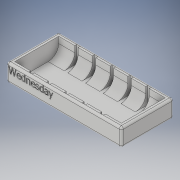
# Autodesk Inventor part: Wednesday
Saved by Autodesk Inventor 2019.4 (Build 234330000, 330)
## iProperties
Created: 2020-10-20
Part Number: Wednesday
Material: Generic
Document SubType Name: Modeling
Designer: daanswinters
Density: 1 g/cm^3
Appearance: Default
Author: daanswinters
Autodesk Inventor part; units mm, degrees
ref_plane "YZ Plane" through (0, 0, 0) normal (1, 0, 0) x (0, 1, 0)
ref_plane "XZ Plane" through (0, 0, 0) normal (0, 1, 0) x (-1, 0, 0)
ref_plane "XY Plane" through (0, 0, 0) normal (0, 0, 1) x (1, 0, 0)
sketch "Sketch1" plane through (0, 0, 0) normal (0, 0, 1) x (1, 0, 0)
  line L0 (55, -8.5) -> (-55, -8.5)
  line L1 (-55, -8.5) -> (-55, 8.5)
  line L2 (-55, 8.5) -> (55, 8.5)
  line L3 (55, 8.5) -> (55, -8.5)
  line L4 (55, -8.5) -> (-55, 8.5) construction
  line L5 (-55, -8.5) -> (55, 8.5) construction
  point P0 (0, 0)
  dimension "d0" = 110
  dimension "d1" = 17
  constraints: 12 end point, 2 midpoint, 2 parallel, 1 horizontal, 1 perpendicular
  measures "d0" distance of L1.end L2.end
  measures "d1" distance of L0.end L1.end
extrude "Extrusion1" add sketch "Sketch1" along normal blind 50
sketch "Sketch2" plane through (-55, 8.5, 0) normal (0, 1, 0) x (1, 0, 0)
  line L0 (0, 0) -> (0, -50) projected
  line L1 (110, -50) -> (0, -50)
  line L2 (0, -50) -> (0, 0)
  line L3 (0, 0) -> (110, 0)
  line L4 (110, 0) -> (110, -50)
  line L5 (110, -50) -> (0, 0) construction
  line L6 (0, -50) -> (110, 0) construction
  line L7 (106, -46) -> (106, -4)
  line L8 (4, -4) -> (4, -46)
  line L9 (56.15, -2) -> (53.85, -2)
  line L10 (53.85, -48) -> (56.15, -48)
  line L11 (56.15, -2) -> (53.85, -48) construction
  line L12 (53.85, -2) -> (56.15, -48) construction
  line L13 (73.15, -2) -> (70.85, -2)
  line L14 (70.85, -48) -> (73.15, -48)
  line L15 (73.15, -2) -> (70.85, -48) construction
  line L16 (70.85, -2) -> (73.15, -48) construction
  line L17 (0, -25) -> (110, -25) construction
  line L18 (87.85, -2) -> (90.15, -2)
  line L19 (90.15, -48) -> (87.85, -48)
  line L20 (87.85, -2) -> (90.15, -48) construction
  line L21 (90.15, -2) -> (87.85, -48) construction
  line L22 (36.85, -2) -> (39.15, -2)
  line L23 (39.15, -48) -> (36.85, -48)
  line L24 (36.85, -2) -> (39.15, -48) construction
  line L25 (39.15, -2) -> (36.85, -48) construction
  line L26 (19.85, -2) -> (22.15, -2)
  line L27 (22.15, -48) -> (19.85, -48)
  line L28 (19.85, -2) -> (22.15, -48) construction
  line L29 (22.15, -2) -> (19.85, -48) construction
  line L30 (90.15, -2) -> (90.15, -4)
  line L31 (90.15, -46) -> (90.15, -48)
  line L32 (87.85, -48) -> (87.85, -46)
  line L33 (87.85, -4) -> (87.85, -2)
  line L34 (73.15, -48) -> (73.15, -46)
  line L35 (73.15, -4) -> (73.15, -2)
  line L36 (70.85, -2) -> (70.85, -4)
  line L37 (70.85, -46) -> (70.85, -48)
  line L38 (56.15, -4) -> (56.15, -2)
  line L39 (53.85, -2) -> (53.85, -4)
  line L40 (53.85, -46) -> (53.85, -48)
  line L41 (56.15, -48) -> (56.15, -46)
  line L42 (39.15, -2) -> (39.15, -4)
  line L43 (39.15, -46) -> (39.15, -48)
  line L44 (36.85, -48) -> (36.85, -46)
  line L45 (36.85, -4) -> (36.85, -2)
  line L46 (22.15, -2) -> (22.15, -4)
  line L47 (19.85, -48) -> (19.85, -46)
  line L48 (19.85, -4) -> (19.85, -2)
  line L49 (22.15, -46) -> (22.15, -48)
  line L50 (4, -46) -> (19.95, -46)
  line L51 (22.05, -46) -> (36.95, -46)
  line L52 (39.05, -46) -> (53.95, -46)
  line L53 (56.05, -46) -> (70.95, -46)
  line L54 (73.05, -46) -> (87.95, -46)
  line L55 (90.05, -46) -> (106, -46)
  line L56 (106, -4) -> (90.05, -4)
  line L57 (87.95, -4) -> (73.05, -4)
  line L58 (70.95, -4) -> (56.05, -4)
  line L59 (53.95, -4) -> (39.05, -4)
  line L60 (36.95, -4) -> (22.05, -4)
  line L61 (19.95, -4) -> (4, -4)
  point P0 (55, 0)
  point P1 (55, -25)
  point P2 (72, -25)
  point P3 (89, -25)
  point P4 (38, -25)
  point P5 (21, -25)
  dimension "d4" = 65.556
  dimension "d5" = 110
  dimension "d7" = 2.3
  dimension "d8" = 46
  dimension "d9" = 2.3
  dimension "d10" = 46
  dimension "d11" = 0
  dimension "d12" = 2.3
  dimension "d13" = 46
  dimension "d14" = 2.3
  dimension "d15" = 46
  dimension "d16" = 2.3
  dimension "d17" = 46
  dimension "d18" = 17
  dimension "d19" = 17
  dimension "d20" = 17
  dimension "d21" = 17
  dimension "d22" = 2.862
  dimension "d23" = 2.862
  dimension "d24" = 106
  dimension "d25" = 4
  dimension "d26" = 42
  dimension "d27" = 2
  dimension "d28" = 0
  dimension "d29" = 42
  dimension "d30" = 0
  dimension "d31" = 42
  dimension "d32" = 0
  dimension "d33" = 42
  dimension "d34" = 0
  dimension "d35" = 42
  dimension "d36" = 0
  dimension "d37" = 42
  constraints: 122 end point, 73 parallel, 43 point on line, 17 perpendicular, 14 midpoint, 6 horizontal
  measures "d4" angle of L5 L0
  measures "d5" distance between parallel lines of L4 L0
  measures "d7" distance of L10.end L10.start
  measures "d8" distance of L10.start L9.end
  measures "d9" distance of L14.end L14.start
  measures "d10" distance of L14.start L13.end
  measures "d11" distance from line of L17 point (72, -25)
  measures "d12" distance of L19.start L19.end
  measures "d13" distance of L18.end L19.start
  measures "d14" distance of L23.start L23.end
  measures "d15" distance of L22.end L23.start
  measures "d16" distance of L27.start L27.end
  measures "d17" distance of L26.end L27.start
  measures "d18" distance of point (72, -25) point (55, -25)
  measures "d19" distance of point (89, -25) point (72, -25)
  measures "d20" distance of point (38, -25) point (55, -25)
  measures "d21" distance of point (21, -25) point (38, -25)
  measures "d22" angle of L0 L20
  measures "d23" angle of L0 L21
  measures "d24" distance between parallel lines of L7 L0
  measures "d25" distance between parallel lines of L8 L0
  measures "d26" distance between parallel lines of L56 L55
  measures "d27" distance between parallel lines of L56 L18
  measures "d28" distance between parallel lines of L56 L57
  measures "d29" distance between parallel lines of L56 L54
  measures "d30" distance between parallel lines of L56 L58
  measures "d31" distance between parallel lines of L56 L53
  measures "d32" distance between parallel lines of L56 L59
  measures "d33" distance between parallel lines of L56 L52
  measures "d34" distance between parallel lines of L56 L60
  measures "d35" distance between parallel lines of L56 L51
  measures "d36" distance between parallel lines of L56 L61
  measures "d37" distance between parallel lines of L56 L50
extrude "Extrusion2" cut sketch "Sketch2" against normal blind 16 contours L55 L31 L19 L32 L54 L34 L14 L37 L53 L41 L10 L40 L52 L43 L23 L44 L51 L49 L27 L47 L50 L8 L61 L48 L26 L46 L60 L45 L22 L42 L59 L39 L9 L38 L58 L36 L13 L35 L57 L33 L18 L30 L56 L7
fillet "Fillet1" radius 2 12 edges at (-55, 0, 50) (-55, 0, 0) (55, 0, 50) (55, 0, 0) (0, 8.5, 50) (-55, 8.5, 25) (0, 8.5, 0) (55, 8.5, 25) (55, -8.5, 25) (0, -8.5, 50) (-55, -8.5, 25) (0, -8.5, 0)
fillet "Fillet2" radius 10 6 edges at (-43.075, -7.5, 4) (-25.5, -7.5, 4) (-8.5, -7.5, 4) (8.5, -7.5, 4) (25.5, -7.5, 4) (43.075, -7.5, 4)
sketch "Sketch3" plane through (35.15, 8.5, 4) normal (0, 1, 0) x (1, 0, 0)
  line L0 (-70.3, -44) -> (-70.3, -42) projected
  line L1 (-51, 2) -> (-53.3, 2)
  line L2 (-34, 2) -> (-34, 0) projected
  line L3 (-36.3, -44) -> (-36.3, -42) projected
  line L4 (-19.3, -44) -> (-19.3, -42) projected
  line L5 (-2.3, -44) -> (-2.3, -42) projected
  line L6 (0, 2) -> (0, 0) projected
  line L7 (-19.8, 2) -> (-16.5, 2)
  line L8 (-16.5, 2) -> (-16.5, -44)
  line L9 (-16.5, -44) -> (-19.8, -44)
  line L10 (-19.8, -44) -> (-19.8, 2)
  line L11 (-19.8, 2) -> (-16.5, -44) construction
  line L12 (-16.5, 2) -> (-19.8, -44) construction
  line L13 (-2.8, -44) -> (0.5, -44)
  line L14 (0.5, -44) -> (0.5, 2)
  line L15 (0.5, 2) -> (-2.8, 2)
  line L16 (-2.8, 2) -> (-2.8, -44)
  line L17 (-2.8, -44) -> (0.5, 2) construction
  line L18 (0.5, -44) -> (-2.8, 2) construction
  line L19 (-36.8, -44) -> (-33.5, -44)
  line L20 (-33.5, -44) -> (-33.5, 2)
  line L21 (-33.5, 2) -> (-36.8, 2)
  line L22 (-36.8, 2) -> (-36.8, -44)
  line L23 (-36.8, -44) -> (-33.5, 2) construction
  line L24 (-33.5, -44) -> (-36.8, 2) construction
  line L25 (-51, 2) -> (-36.3, 2) projected
  line L26 (-53.8, -44) -> (-50.5, -44)
  line L27 (-50.5, -44) -> (-50.5, 2)
  line L28 (-50.5, 2) -> (-53.8, 2)
  line L29 (-53.8, 2) -> (-53.8, -44)
  line L30 (-53.8, -44) -> (-50.5, 2) construction
  line L31 (-50.5, -44) -> (-53.8, 2) construction
  line L32 (-53.3, -44) -> (-68, -44) projected
  line L33 (-70.8, 2) -> (-67.5, 2)
  line L34 (-67.5, 2) -> (-67.5, -44)
  line L35 (-67.5, -44) -> (-70.8, -44)
  line L36 (-70.8, -44) -> (-70.8, 2)
  line L37 (-70.8, 2) -> (-67.5, -44) construction
  line L38 (-67.5, 2) -> (-70.8, -44) construction
  point P0 (-35.15, 4)
  point P1 (-68, 2)
  point P2 (-17, 2)
  point P3 (-18.15, -21)
  point P4 (-1.15, -21)
  point P5 (-35.15, -21)
  point P6 (-52.15, -21)
  point P7 (-69.15, -21)
  dimension "d42" = 3.3
  dimension "d43" = 46
  dimension "d44" = 3.3
  dimension "d45" = 3.3
  dimension "d46" = 3.3
  dimension "d47" = 3.3
  dimension "d48" = 90
  dimension "d49" = 0.5
  dimension "d50" = 16.5
  dimension "d51" = 33.5
  dimension "d52" = 50.5
  dimension "d53" = 67.5
  dimension "d54" = 46
  dimension "d55" = 0
  dimension "d56" = 53.3
  constraints: 62 end point, 14 parallel, 10 midpoint, 5 horizontal, 5 perpendicular, 3 point on line
  measures "d42" distance of L8.end L9.end
  measures "d43" distance of L7.end L8.end
  measures "d44" distance of L15.end L14.end
  measures "d45" distance of L21.end L20.end
  measures "d46" distance of L28.end L27.end
  measures "d47" distance of L34.end L35.end
  measures "d48" angle of L6 L1
  measures "d49" distance between parallel lines of L6 L14
  measures "d50" distance between parallel lines of L6 L8
  measures "d51" distance between parallel lines of L6 L20
  measures "d52" distance between parallel lines of L6 L27
  measures "d53" distance between parallel lines of L6 L34
  measures "d54" distance between parallel lines of L25 L9
  measures "d55" distance between parallel lines of L15 L25
  measures "d56" distance from line of L1.end L6
extrude "Extrusion3" cut sketch "Sketch3" against normal blind 16
sketch "Sketch4" plane through (0, 0, 50) normal (0, 0, 1) x (1, 0, 0)
  line L0 (-52.9749, 6.5012) -> (53.0345, 6.5012) construction
  line L1 (53.0345, 6.5012) -> (53.0345, -6.5247) construction
  line L2 (53.0345, -6.5247) -> (-52.9749, -6.5247) construction
  line L3 (-52.9749, -6.5247) -> (-52.9749, 6.5012) construction
  line L4 (-45.5205, 6.2294) -> (-47.0529, 0.1294)
  line L5 (-47.0529, 0.1294) -> (-47.9624, 0.1294)
  line L6 (-47.9624, 0.1294) -> (-49.2032, 5.1913)
  line L7 (-49.2032, 5.1913) -> (-50.4094, 0.1294)
  line L8 (-50.4094, 0.1294) -> (-51.309, 0.1294)
  line L9 (-51.309, 0.1294) -> (-52.8662, 6.2294)
  line L10 (-52.8662, 6.2294) -> (-52.0308, 6.2294)
  line L11 (-52.0308, 6.2294) -> (-50.8048, 1.1724)
  line L12 (-50.8048, 1.1724) -> (-49.5888, 6.2294)
  line L13 (-49.5888, 6.2294) -> (-48.7633, 6.2294)
  line L14 (-48.7633, 6.2294) -> (-47.5373, 1.1131)
  line L15 (-47.5373, 1.1131) -> (-46.3163, 6.2294)
  line L16 (-46.3163, 6.2294) -> (-45.5205, 6.2294)
  spline S0 degree 2 poles (-42.8659, 0.0256) (-43.9633, 0.0256) (-45.1695, 1.2564) (-45.1695, 2.3934) knots 0 0 0 1 2 2 2
  spline S1 degree 2 poles (-45.1695, 2.3934) (-45.1695, 3.5106) (-43.9979, 4.8354) (-43.0538, 4.8354) knots 0 0 0 1 2 2 2
  spline S2 degree 2 poles (-43.0538, 4.8354) (-42.6287, 4.8354) (-41.9712, 4.5882) (-41.729, 4.3262) knots 0 0 0 1 2 2 2
  spline S3 degree 2 poles (-41.729, 4.3262) (-41.4818, 4.0642) (-41.2198, 3.3079) (-41.2198, 2.7592) knots 0 0 0 1 2 2 2
  line L17 (-41.2198, 2.7592) -> (-41.2198, 2.339)
  line L18 (-41.2198, 2.339) -> (-44.3885, 2.339)
  spline S4 degree 2 poles (-44.3885, 2.339) (-44.3885, 1.5431) (-43.5876, 0.6978) (-42.8758, 0.6978) knots 0 0 0 1 2 2 2
  spline S5 degree 2 poles (-42.8758, 0.6978) (-42.6237, 0.6978) (-42.1343, 0.8115) (-41.9366, 0.9005) knots 0 0 0 1 2 2 2
  spline S6 degree 2 poles (-41.9366, 0.9005) (-41.729, 0.9994) (-41.4423, 1.1724) (-41.3483, 1.2515) knots 0 0 0 1 2 2 2
  line L19 (-41.3483, 1.2515) -> (-41.3039, 1.2515)
  line L20 (-41.3039, 1.2515) -> (-41.3039, 0.4111)
  spline S7 degree 2 poles (-41.3039, 0.4111) (-41.4373, 0.3568) (-41.8427, 0.1986) (-42.0009, 0.1541) knots 0 0 0 1 2 2 2
  spline S8 degree 2 poles (-42.0009, 0.1541) (-42.2233, 0.0898) (-42.5891, 0.0256) (-42.8659, 0.0256) knots 0 0 0 1 2 2 2
  spline S9 degree 2 poles (-41.9712, 2.9273) (-41.9811, 3.2387) (-42.1096, 3.6935) (-42.2332, 3.8467) knots 0 0 0 1 2 2 2
  spline S10 degree 2 poles (-42.2332, 3.8467) (-42.3667, 4.0197) (-42.7868, 4.2026) (-43.0983, 4.2026) knots 0 0 0 1 2 2 2
  spline S11 degree 2 poles (-43.0983, 4.2026) (-43.4047, 4.2026) (-43.8348, 4.0197) (-44.0128, 3.8418) knots 0 0 0 1 2 2 2
  spline S12 degree 2 poles (-44.0128, 3.8418) (-44.1858, 3.6589) (-44.3637, 3.2189) (-44.3885, 2.9273) knots 0 0 0 1 2 2 2
  line L21 (-44.3885, 2.9273) -> (-41.9712, 2.9273)
  line L22 (-36.9192, 0.1294) -> (-37.6903, 0.1294)
  line L23 (-37.6903, 0.1294) -> (-37.6903, 0.594)
  spline S13 degree 2 poles (-37.6903, 0.594) (-37.8683, 0.4457) (-38.1303, 0.248) (-38.3082, 0.164) knots 0 0 0 1 2 2 2
  spline S14 degree 2 poles (-38.3082, 0.164) (-38.4714, 0.0849) (-38.8223, 0.0008) (-39.0547, 0.0008) knots 0 0 0 1 2 2 2
  spline S15 degree 2 poles (-39.0547, 0.0008) (-39.4304, 0.0008) (-40.0631, 0.3123) (-40.2855, 0.6138) knots 0 0 0 1 2 2 2
  spline S16 degree 2 poles (-40.2855, 0.6138) (-40.508, 0.9153) (-40.7552, 1.8051) (-40.7552, 2.3835) knots 0 0 0 1 2 2 2
  spline S17 degree 2 poles (-40.7552, 2.3835) (-40.7552, 2.9866) (-40.4437, 3.8665) (-40.1718, 4.1977) knots 0 0 0 1 2 2 2
  spline S18 degree 2 poles (-40.1718, 4.1977) (-39.9197, 4.4943) (-39.2129, 4.8354) (-38.8223, 4.8354) knots 0 0 0 1 2 2 2
  spline S19 degree 2 poles (-38.8223, 4.8354) (-38.4812, 4.8354) (-37.9721, 4.6821) (-37.6903, 4.5239) knots 0 0 0 1 2 2 2
  line L24 (-37.6903, 4.5239) -> (-37.6903, 6.5012)
  line L25 (-37.6903, 6.5012) -> (-36.9192, 6.5012)
  line L26 (-36.9192, 6.5012) -> (-36.9192, 0.1294)
  line L27 (-37.6903, 1.2416) -> (-37.6903, 3.8863)
  spline S20 degree 2 poles (-37.6903, 3.8863) (-37.977, 4.0247) (-38.4318, 4.1285) (-38.6938, 4.1285) knots 0 0 0 1 2 2 2
  spline S21 degree 2 poles (-38.6938, 4.1285) (-39.287, 4.1285) (-39.9593, 3.2387) (-39.9593, 2.3983) knots 0 0 0 1 2 2 2
  spline S22 degree 2 poles (-39.9593, 2.3983) (-39.9593, 1.5876) (-39.4452, 0.7324) (-38.8767, 0.7324) knots 0 0 0 1 2 2 2
  spline S23 degree 2 poles (-38.8767, 0.7324) (-38.5752, 0.7324) (-37.9622, 1.0093) (-37.6903, 1.2416) knots 0 0 0 1 2 2 2
  line L28 (-32.2082, 0.1294) -> (-32.9794, 0.1294)
  line L29 (-32.9794, 0.1294) -> (-32.9794, 2.7394)
  spline S24 degree 2 poles (-32.9794, 2.7394) (-32.9794, 3.0558) (-33.0387, 3.5995) (-33.1277, 3.7627) knots 0 0 0 1 2 2 2
  spline S25 degree 2 poles (-33.1277, 3.7627) (-33.2216, 3.9357) (-33.5577, 4.1038) (-33.8445, 4.1038) knots 0 0 0 1 2 2 2
  spline S26 degree 2 poles (-33.8445, 4.1038) (-34.1312, 4.1038) (-34.7392, 3.7973) (-35.0308, 3.5501) knots 0 0 0 1 2 2 2
  line L30 (-35.0308, 3.5501) -> (-35.0308, 0.1294)
  line L31 (-35.0308, 0.1294) -> (-35.802, 0.1294)
  line L32 (-35.802, 0.1294) -> (-35.802, 4.7068)
  line L33 (-35.802, 4.7068) -> (-35.0308, 4.7068)
  line L34 (-35.0308, 4.7068) -> (-35.0308, 4.1977)
  spline S27 degree 2 poles (-35.0308, 4.1977) (-34.6848, 4.5091) (-34.0175, 4.8354) (-33.6418, 4.8354) knots 0 0 0 1 2 2 2
  spline S28 degree 2 poles (-33.6418, 4.8354) (-32.9695, 4.8354) (-32.2082, 3.9456) (-32.2082, 3.1003) knots 0 0 0 1 2 2 2
  line L35 (-32.2082, 3.1003) -> (-32.2082, 0.1294)
  spline S29 degree 2 poles (-29.1385, 0.0256) (-30.2359, 0.0256) (-31.442, 1.2564) (-31.442, 2.3934) knots 0 0 0 1 2 2 2
  spline S30 degree 2 poles (-31.442, 2.3934) (-31.442, 3.5106) (-30.2705, 4.8354) (-29.3263, 4.8354) knots 0 0 0 1 2 2 2
  spline S31 degree 2 poles (-29.3263, 4.8354) (-28.9012, 4.8354) (-28.2437, 4.5882) (-28.0015, 4.3262) knots 0 0 0 1 2 2 2
  spline S32 degree 2 poles (-28.0015, 4.3262) (-27.7543, 4.0642) (-27.4923, 3.3079) (-27.4923, 2.7592) knots 0 0 0 1 2 2 2
  line L36 (-27.4923, 2.7592) -> (-27.4923, 2.339)
  line L37 (-27.4923, 2.339) -> (-30.661, 2.339)
  spline S33 degree 2 poles (-30.661, 2.339) (-30.661, 1.5431) (-29.8602, 0.6978) (-29.1483, 0.6978) knots 0 0 0 1 2 2 2
  spline S34 degree 2 poles (-29.1483, 0.6978) (-28.8962, 0.6978) (-28.4069, 0.8115) (-28.2091, 0.9005) knots 0 0 0 1 2 2 2
  spline S35 degree 2 poles (-28.2091, 0.9005) (-28.0015, 0.9994) (-27.7148, 1.1724) (-27.6209, 1.2515) knots 0 0 0 1 2 2 2
  line L38 (-27.6209, 1.2515) -> (-27.5764, 1.2515)
  line L39 (-27.5764, 1.2515) -> (-27.5764, 0.4111)
  spline S36 degree 2 poles (-27.5764, 0.4111) (-27.7099, 0.3568) (-28.1152, 0.1986) (-28.2734, 0.1541) knots 0 0 0 1 2 2 2
  spline S37 degree 2 poles (-28.2734, 0.1541) (-28.4958, 0.0898) (-28.8616, 0.0256) (-29.1385, 0.0256) knots 0 0 0 1 2 2 2
  spline S38 degree 2 poles (-28.2437, 2.9273) (-28.2536, 3.2387) (-28.3821, 3.6935) (-28.5057, 3.8467) knots 0 0 0 1 2 2 2
  spline S39 degree 2 poles (-28.5057, 3.8467) (-28.6392, 4.0197) (-29.0594, 4.2026) (-29.3708, 4.2026) knots 0 0 0 1 2 2 2
  spline S40 degree 2 poles (-29.3708, 4.2026) (-29.6773, 4.2026) (-30.1073, 4.0197) (-30.2853, 3.8418) knots 0 0 0 1 2 2 2
  spline S41 degree 2 poles (-30.2853, 3.8418) (-30.4583, 3.6589) (-30.6363, 3.2189) (-30.661, 2.9273) knots 0 0 0 1 2 2 2
  line L40 (-30.661, 2.9273) -> (-28.2437, 2.9273)
  spline S42 degree 2 poles (-25.4755, 0.0206) (-25.9352, 0.0206) (-26.7311, 0.2678) (-26.9931, 0.4062) knots 0 0 0 1 2 2 2
  line L41 (-26.9931, 0.4062) -> (-26.9931, 1.2713)
  line L42 (-26.9931, 1.2713) -> (-26.9535, 1.2713)
  spline S43 degree 2 poles (-26.9535, 1.2713) (-26.8547, 1.1922) (-26.5877, 1.0043) (-26.3653, 0.9005) knots 0 0 0 1 2 2 2
  spline S44 degree 2 poles (-26.3653, 0.9005) (-26.1725, 0.8066) (-25.6979, 0.6682) (-25.4458, 0.6682) knots 0 0 0 1 2 2 2
  spline S45 degree 2 poles (-25.4458, 0.6682) (-25.2629, 0.6682) (-24.8428, 0.7522) (-24.7439, 0.8214) knots 0 0 0 1 2 2 2
  spline S46 degree 2 poles (-24.7439, 0.8214) (-24.6005, 0.9153) (-24.472, 1.1279) (-24.472, 1.3454) knots 0 0 0 1 2 2 2
  spline S47 degree 2 poles (-24.472, 1.3454) (-24.472, 1.6173) (-24.7686, 1.8991) (-25.1492, 1.993) knots 0 0 0 1 2 2 2
  spline S48 degree 2 poles (-25.1492, 1.993) (-25.2975, 2.0276) (-25.7721, 2.1265) (-25.9748, 2.1808) knots 0 0 0 1 2 2 2
  spline S49 degree 2 poles (-25.9748, 2.1808) (-26.4988, 2.3341) (-26.9733, 2.9668) (-26.9733, 3.4166) knots 0 0 0 1 2 2 2
  spline S50 degree 2 poles (-26.9733, 3.4166) (-26.9733, 4.0395) (-26.039, 4.8156) (-25.2679, 4.8156) knots 0 0 0 1 2 2 2
  spline S51 degree 2 poles (-25.2679, 4.8156) (-24.8872, 4.8156) (-24.1161, 4.6277) (-23.8541, 4.4844) knots 0 0 0 1 2 2 2
  line L43 (-23.8541, 4.4844) -> (-23.8541, 3.6589)
  line L44 (-23.8541, 3.6589) -> (-23.8936, 3.6589)
  spline S52 degree 2 poles (-23.8936, 3.6589) (-24.1902, 3.8961) (-24.912, 4.168) (-25.2827, 4.168) knots 0 0 0 1 2 2 2
  spline S53 degree 2 poles (-25.2827, 4.168) (-25.6633, 4.168) (-26.1873, 3.8467) (-26.1873, 3.5254) knots 0 0 0 1 2 2 2
  spline S54 degree 2 poles (-26.1873, 3.5254) (-26.1873, 3.2337) (-25.8759, 2.952) (-25.5299, 2.863) knots 0 0 0 1 2 2 2
  spline S55 degree 2 poles (-25.5299, 2.863) (-25.3618, 2.8185) (-24.9367, 2.7295) (-24.7043, 2.6752) knots 0 0 0 1 2 2 2
  spline S56 degree 2 poles (-24.7043, 2.6752) (-24.2001, 2.5466) (-23.686, 1.9584) (-23.686, 1.4492) knots 0 0 0 1 2 2 2
  spline S57 degree 2 poles (-23.686, 1.4492) (-23.686, 1.1526) (-23.9184, 0.6286) (-24.1458, 0.4359) knots 0 0 0 1 2 2 2
  spline S58 degree 2 poles (-24.1458, 0.4359) (-24.388, 0.2332) (-25.0059, 0.0206) (-25.4755, 0.0206) knots 0 0 0 1 2 2 2
  line L45 (-19.4496, 0.1294) -> (-20.2208, 0.1294)
  line L46 (-20.2208, 0.1294) -> (-20.2208, 0.594)
  spline S59 degree 2 poles (-20.2208, 0.594) (-20.3988, 0.4457) (-20.6607, 0.248) (-20.8387, 0.164) knots 0 0 0 1 2 2 2
  spline S60 degree 2 poles (-20.8387, 0.164) (-21.0018, 0.0849) (-21.3528, 0.0008) (-21.5851, 0.0008) knots 0 0 0 1 2 2 2
  spline S61 degree 2 poles (-21.5851, 0.0008) (-21.9608, 0.0008) (-22.5936, 0.3123) (-22.816, 0.6138) knots 0 0 0 1 2 2 2
  spline S62 degree 2 poles (-22.816, 0.6138) (-23.0385, 0.9153) (-23.2856, 1.8051) (-23.2856, 2.3835) knots 0 0 0 1 2 2 2
  spline S63 degree 2 poles (-23.2856, 2.3835) (-23.2856, 2.9866) (-22.9742, 3.8665) (-22.7023, 4.1977) knots 0 0 0 1 2 2 2
  spline S64 degree 2 poles (-22.7023, 4.1977) (-22.4502, 4.4943) (-21.7433, 4.8354) (-21.3528, 4.8354) knots 0 0 0 1 2 2 2
  spline S65 degree 2 poles (-21.3528, 4.8354) (-21.0117, 4.8354) (-20.5026, 4.6821) (-20.2208, 4.5239) knots 0 0 0 1 2 2 2
  line L47 (-20.2208, 4.5239) -> (-20.2208, 6.5012)
  line L48 (-20.2208, 6.5012) -> (-19.4496, 6.5012)
  line L49 (-19.4496, 6.5012) -> (-19.4496, 0.1294)
  line L50 (-20.2208, 1.2416) -> (-20.2208, 3.8863)
  spline S66 degree 2 poles (-20.2208, 3.8863) (-20.5075, 4.0247) (-20.9623, 4.1285) (-21.2243, 4.1285) knots 0 0 0 1 2 2 2
  spline S67 degree 2 poles (-21.2243, 4.1285) (-21.8175, 4.1285) (-22.4898, 3.2387) (-22.4898, 2.3983) knots 0 0 0 1 2 2 2
  spline S68 degree 2 poles (-22.4898, 2.3983) (-22.4898, 1.5876) (-21.9757, 0.7324) (-21.4072, 0.7324) knots 0 0 0 1 2 2 2
  spline S69 degree 2 poles (-21.4072, 0.7324) (-21.1056, 0.7324) (-20.4927, 1.0093) (-20.2208, 1.2416) knots 0 0 0 1 2 2 2
  spline S70 degree 2 poles (-15.7817, 0.6138) (-15.8757, 0.5446) (-16.192, 0.2974) (-16.3403, 0.2233) knots 0 0 0 1 2 2 2
  spline S71 degree 2 poles (-16.3403, 0.2233) (-16.543, 0.1145) (-16.9236, 0.0008) (-17.2697, 0.0008) knots 0 0 0 1 2 2 2
  spline S72 degree 2 poles (-17.2697, 0.0008) (-17.5514, 0.0008) (-18.0606, 0.2134) (-18.2534, 0.4062) knots 0 0 0 1 2 2 2
  spline S73 degree 2 poles (-18.2534, 0.4062) (-18.4363, 0.594) (-18.6587, 1.1477) (-18.6587, 1.4542) knots 0 0 0 1 2 2 2
  spline S74 degree 2 poles (-18.6587, 1.4542) (-18.6587, 1.9287) (-18.2583, 2.601) (-17.8233, 2.7938) knots 0 0 0 1 2 2 2
  spline S75 degree 2 poles (-17.8233, 2.7938) (-17.4377, 2.9718) (-16.3898, 3.1052) (-15.7817, 3.1398) knots 0 0 0 1 2 2 2
  line L51 (-15.7817, 3.1398) -> (-15.7817, 3.2881)
  spline S76 degree 2 poles (-15.7817, 3.2881) (-15.7817, 3.5551) (-15.9449, 3.8863) (-16.0932, 3.9802) knots 0 0 0 1 2 2 2
  spline S77 degree 2 poles (-16.0932, 3.9802) (-16.2415, 4.0741) (-16.6666, 4.1334) (-16.894, 4.1334) knots 0 0 0 1 2 2 2
  spline S78 degree 2 poles (-16.894, 4.1334) (-17.1609, 4.1334) (-17.8826, 3.9752) (-18.2435, 3.822) knots 0 0 0 1 2 2 2
  line L52 (-18.2435, 3.822) -> (-18.288, 3.822)
  line L53 (-18.288, 3.822) -> (-18.288, 4.608)
  spline S79 degree 2 poles (-18.288, 4.608) (-18.0754, 4.6673) (-17.2795, 4.8156) (-16.889, 4.8156) knots 0 0 0 1 2 2 2
  spline S80 degree 2 poles (-16.889, 4.8156) (-16.4145, 4.8156) (-15.7669, 4.6673) (-15.5099, 4.4745) knots 0 0 0 1 2 2 2
  spline S81 degree 2 poles (-15.5099, 4.4745) (-15.2577, 4.2867) (-15.0106, 3.6885) (-15.0106, 3.2585) knots 0 0 0 1 2 2 2
  line L54 (-15.0106, 3.2585) -> (-15.0106, 0.1294)
  line L55 (-15.0106, 0.1294) -> (-15.7817, 0.1294)
  line L56 (-15.7817, 0.1294) -> (-15.7817, 0.6138)
  line L57 (-15.7817, 1.2564) -> (-15.7817, 2.5269)
  spline S82 degree 2 poles (-15.7817, 2.5269) (-16.0586, 2.5021) (-16.894, 2.4181) (-17.156, 2.339) knots 0 0 0 1 2 2 2
  spline S83 degree 2 poles (-17.156, 2.339) (-17.4624, 2.2451) (-17.8629, 1.8546) (-17.8629, 1.5085) knots 0 0 0 1 2 2 2
  spline S84 degree 2 poles (-17.8629, 1.5085) (-17.8629, 1.1131) (-17.418, 0.7127) (-16.9928, 0.7127) knots 0 0 0 1 2 2 2
  spline S85 degree 2 poles (-16.9928, 0.7127) (-16.632, 0.7127) (-16.0388, 1.0241) (-15.7817, 1.2564) knots 0 0 0 1 2 2 2
  line L58 (-10.3342, 4.7068) -> (-12.796, -1.5563)
  line L59 (-12.796, -1.5563) -> (-13.6215, -1.5563)
  line L60 (-13.6215, -1.5563) -> (-12.8009, 0.3518)
  line L61 (-12.8009, 0.3518) -> (-14.4619, 4.7068)
  line L62 (-14.4619, 4.7068) -> (-13.6314, 4.7068)
  line L63 (-13.6314, 4.7068) -> (-12.3808, 1.3158)
  line L64 (-12.3808, 1.3158) -> (-11.1351, 4.7068)
  line L65 (-11.1351, 4.7068) -> (-10.3342, 4.7068)
  point P0 (0, 0)
  constraints: 2 other
extrude "Extrusion4" cut sketch "Sketch4" against normal blind 0.5
fillet "Fillet3" radius 10 6 edges at (-43.325, -7.5, 46) (-25.5, -7.5, 46) (-8.5, -7.5, 46) (8.5, -7.5, 46) (25.5, -7.5, 46) (43.325, -7.5, 46)
body "Solid1"
